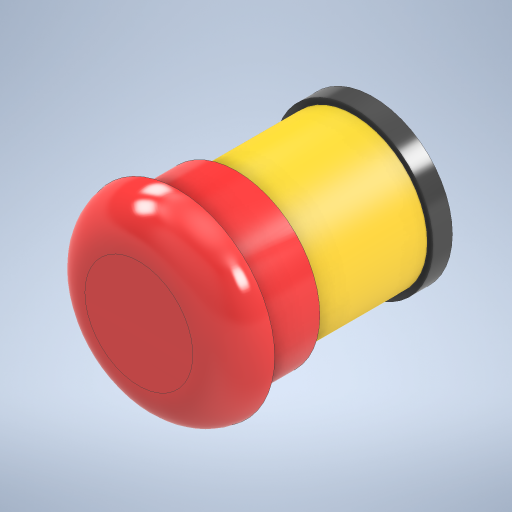
# Autodesk Inventor part: hitan_stop
Saved by Autodesk Inventor 2023 (Build 270158000, 158)
## iProperties
Created: 2022-07-17
Part Number: hitan_stop
Material: Generic
Document SubType Name: Sheet Metal
Designer: User
Density: 1 g/cm^3
Sheet Metal Rule: Default
Appearance: Default
Author: User
Autodesk Inventor part; units mm, degrees
ref_plane "YZ Plane" through (0, 0, 0) normal (1, 0, 0) x (0, 1, 0)
ref_plane "XZ Plane" through (0, 0, 0) normal (0, 1, 0) x (-1, 0, 0)
ref_plane "XY Plane" through (0, 0, 0) normal (0, 0, 1) x (1, 0, 0)
sketch "Sketch1" plane through (0, 0, 0) normal (0, 0, 1) x (1, 0, 0)
  circle A0 centre (0, 0) radius 20.32
  dimension "d0" = 40.64
  constraints: 1 centre point, 1 coincident
  measures "d0" diameter of A0
extrude "Extrusion1" add sketch "Sketch1" along normal blind 5
sketch "Sketch2" plane through (0, 0, 5) normal (0, 0, 1) x (1, 0, 0)
  circle A0 centre (0, 0) radius 18.8864
  constraints: 1 centre point
extrude "Extrusion4" add sketch "Sketch2" along normal blind 30
sketch "Sketch3" plane through (0, 0, 35) normal (0, 0, 1) x (1, 0, 0)
  circle A0 centre (0, 0) radius 21.3705
  constraints: 1 centre point, 1 coincident
extrude "Extrusion5" add sketch "Sketch3" along normal blind 15
sketch "Sketch4" plane through (0, 0, 50) normal (0, 0, 1) x (1, 0, 0)
  circle A0 centre (0, 0) radius 24.7853
  constraints: 1 centre point, 1 coincident
extrude "Extrusion6" add sketch "Sketch4" along normal blind 10
fillet "Fillet1" radius 11 1 edges at (-24.7853, 0, 60)
equation "\"BendRadius\" = Thickness"
equation "\"BendReliefWidth\" = Thickness"
equation "\"BendReliefDepth\" = 0.5 * Thickness"
equation "\"CornerReliefSize\" = 4 * Thickness"
equation "\"MinimumRemnant\" = 2 * Thickness"
equation "\"TransitionRadius\" = BendRadius"
equation "\"JacobiRadiusSize\" = BendRadius"
equation "\"GapSize\" = Thickness"
equation "\"Thickness\" = 3.048"
body "Solid1"
